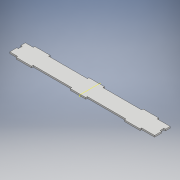
# Autodesk Inventor part: F6
Saved by Autodesk Inventor 2018 (Build 220112000, 112)
## iProperties
Created: 2018-03-06
Part Number: F6
Material: Generic
Document SubType Name: Modeling
Designer: isai
Density: 1 g/cm^3
Appearance: Default
Author: isai
Autodesk Inventor part; units mm, degrees
ref_plane "YZ Plane" through (0, 0, 0) normal (1, 0, 0) x (0, 1, 0)
ref_plane "XZ Plane" through (0, 0, 0) normal (0, 1, 0) x (-1, 0, 0)
ref_plane "XY Plane" through (0, 0, 0) normal (0, 0, 1) x (1, 0, 0)
sketch "Sketch2" plane through (0, 0, 0) normal (0, 0, 1) x (1, 0, 0)
  line L0 (-469, -128.2) -> (-449, -128.2)
  line L1 (-449, -128.2) -> (-449, -124.2)
  line L2 (-449, -124.2) -> (-409, -124.2)
  line L3 (-409, -124.2) -> (-409, -128.2)
  line L4 (-409, -128.2) -> (-309.6667, -128.2)
  line L5 (-309.6667, -128.2) -> (-309.6667, -124.2)
  line L6 (-309.6667, -124.2) -> (-269.6667, -124.2)
  line L7 (-269.6667, -124.2) -> (-269.6667, -128.2)
  line L8 (-269.6667, -128.2) -> (-170.3333, -128.2)
  line L9 (-170.3333, -128.2) -> (-170.3333, -124.2)
  line L10 (-170.3333, -124.2) -> (-130.3333, -124.2)
  line L11 (-130.3333, -124.2) -> (-130.3333, -128.2)
  line L12 (-130.3333, -128.2) -> (-101, -128.2)
  line L13 (-101, -128.2) -> (-97, -128.2)
  line L14 (-97, -128.2) -> (-97, -168.2)
  line L15 (-469, -128.2) -> (-469, -168.2)
  line L16 (-469, -148.2) -> (-513.1523, -148.2)
  line L17 (-170.3333, -168.2) -> (-170.3333, -172.2)
  line L18 (-309.6667, -168.2) -> (-309.6667, -172.2)
  line L19 (-130.3333, -172.2) -> (-130.3333, -168.2)
  line L20 (-449, -172.2) -> (-409, -172.2)
  line L21 (-449, -168.2) -> (-449, -172.2)
  line L22 (-409, -172.2) -> (-409, -168.2)
  line L23 (-269.6667, -172.2) -> (-269.6667, -168.2)
  line L24 (-309.6667, -172.2) -> (-269.6667, -172.2)
  line L25 (-170.3333, -172.2) -> (-130.3333, -172.2)
  line L26 (-449, -168.2) -> (-469, -168.2)
  line L27 (-309.6667, -168.2) -> (-409, -168.2)
  line L28 (-97, -168.2) -> (-130.3333, -168.2)
  line L29 (-170.3333, -168.2) -> (-269.6667, -168.2)
  point P0 (0, 0)
  dimension "d2" = 4
  dimension "d3" = 40
  constraints: 60 end point, 12 symmetric about line, 5 perpendicular, 2 horizontal, 1 midpoint, 1 vertical
  measures "d2" distance of L12.end L13.end
  measures "d3" distance of L13.end L14.end
extrude "Extrusion2" add sketch "Sketch2" along normal blind 4
sketch "Sketch4" plane through (0, 0, 4) normal (0, 0, 1) x (1, 0, 0)
  line L0 (-170.3333, -128.2) -> (-269.6667, -128.2) projected
  line L1 (-269.6667, -128.2) -> (-269.6667, -124.2) projected
  line L2 (-269.6667, -124.2) -> (-309.6667, -124.2) projected
  line L3 (-309.6667, -124.2) -> (-309.6667, -128.2) projected
  line L4 (-309.6667, -128.2) -> (-409, -128.2) projected
  line L5 (-409, -128.2) -> (-409, -124.2) projected
  line L6 (-409, -124.2) -> (-449, -124.2) projected
  line L7 (-449, -124.2) -> (-449, -128.2) projected
  line L8 (-449, -128.2) -> (-469, -128.2) projected
  line L9 (-469, -128.2) -> (-469, -168.2) projected
  line L10 (-469, -168.2) -> (-449, -168.2) projected
  line L11 (-449, -168.2) -> (-449, -172.2) projected
  line L12 (-449, -172.2) -> (-409, -172.2) projected
  line L13 (-409, -172.2) -> (-409, -168.2) projected
  line L14 (-409, -168.2) -> (-309.6667, -168.2) projected
  line L15 (-309.6667, -168.2) -> (-309.6667, -172.2) projected
  line L16 (-309.6667, -172.2) -> (-269.6667, -172.2) projected
  line L17 (-269.6667, -172.2) -> (-269.6667, -168.2) projected
  line L18 (-269.6667, -168.2) -> (-170.3333, -168.2) projected
  line L19 (-170.3333, -168.2) -> (-170.3333, -172.2) projected
  line L20 (-170.3333, -172.2) -> (-130.3333, -172.2) projected
  line L21 (-130.3333, -172.2) -> (-130.3333, -168.2) projected
  line L22 (-130.3333, -168.2) -> (-97, -168.2) projected
  line L23 (-97, -168.2) -> (-97, -128.2) projected
  line L24 (-97, -128.2) -> (-130.3333, -128.2) projected
  line L25 (-130.3333, -128.2) -> (-130.3333, -124.2) projected
  line L26 (-130.3333, -124.2) -> (-170.3333, -124.2) projected
  line L27 (-170.3333, -124.2) -> (-170.3333, -128.2) projected
  line L28 (-469, -140.2844) -> (-465, -140.2844)
  line L29 (-465, -140.2844) -> (-465, -150.2844)
  line L30 (-465, -150.2844) -> (-469, -150.2844)
  line L31 (-469, -150.2844) -> (-469, -140.2844)
  line L32 (-469, -128.2) -> (-469, -168.2) projected
  point P0 (0, 0)
  point P1 (-469, -145.2844)
  dimension "d13" = 4
  dimension "d14" = 10
  constraints: 8 end point, 2 parallel, 1 horizontal, 1 midpoint, 1 perpendicular, 1 point on line
  measures "d13" distance of L29.end L30.end
  measures "d14" distance of L28.end L29.end
extrude "Extrusion4" cut sketch "Sketch4" against normal blind 4 contours L28 L29 L30 L9
ref_plane "Work Plane1" through (-283, -128.2, 0) normal (-1, 0, 0) x (0, 0, 1)
mirror "Mirror1" about plane through (-283, -128.2, 0) normal (-1, 0, 0) of "Extrusion4"
body "Solid2"
